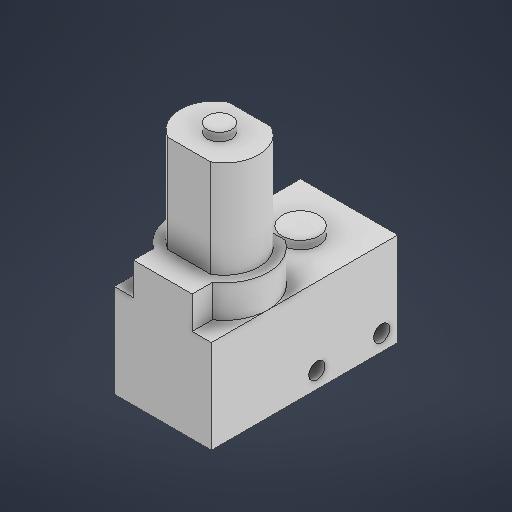
# Autodesk Inventor part: Encoder Motor
Saved by Autodesk Inventor 2026.1 (Build 301233020, 233B)
## iProperties
Created: 2025-10-23
Part Number: Encoder Motor
Material: Generic
Document SubType Name: Modeling
Designer: Asus
Density: 1 g/cm^3
Appearance: Default
Author: Asus
Autodesk Inventor part; units mm, degrees
ref_plane "YZ Plane" through (0, 0, 0) normal (1, 0, 0) x (0, 1, 0)
ref_plane "XZ Plane" through (0, 0, 0) normal (0, 1, 0) x (-1, 0, 0)
ref_plane "XY Plane" through (0, 0, 0) normal (0, 0, 1) x (1, 0, 0)
sketch "Sketch1" plane through (0, 0, 0) normal (0, 1, 0) x (-1, 0, 0)
  line L0 (0, 0) -> (-24, 0)
  line L1 (-24, 0) -> (-24, -46)
  line L2 (-24, -46) -> (0, -46)
  line L3 (0, -46) -> (0, 0)
  dimension "d0" = 24
  dimension "d1" = 46
  constraints: 8 end point, 2 parallel, 1 coincident, 1 horizontal, 1 perpendicular
  measures "d0" distance of L2.end L1.end
  measures "d1" distance of L1.end L0.end
extrude "Extrusion1" add sketch "Sketch1" along normal blind 23
sketch "Sketch2" plane through (0, 23, 0) normal (0, 1, 0) x (1, 0, 0)
  line L0 (4.75, 0) -> (19.25, 0)
  line L1 (19.25, 0) -> (19.25, 5)
  line L2 (19.25, 23) -> (4.75, 23)
  line L3 (4.75, 5) -> (4.75, 0)
  line L4 (4.75, 0) -> (19.25, 23) construction
  line L5 (19.25, 0) -> (4.75, 23) construction
  line L6 (0, 0) -> (24, 0) projected
  arc A0 (13, 23) -> (11, 23) centre (12, 23) ccw
  arc A1 (4.75, 23) -> (4.75, 5) centre (10.9013, 14) ccw
  line L7 (0, 46) -> (0, 0) projected
  arc A2 (19.25, 5) -> (19.25, 23) centre (13.0987, 14) ccw
  line L8 (24, 0) -> (24, 46) projected
  circle A3 centre (12, 34) radius 4.5
  line L9 (24, 46) -> (0, 46) projected
  point P0 (12, 11.5)
  point P1 (12, 0)
  dimension "d4" = 14.5
  dimension "d5" = 23
  dimension "d6" = 2
  dimension "d8" = 9
  dimension "d9" = 12
  constraints: 12 end point, 6 point on circle, 5 midpoint, 4 centre point, 2 parallel, 2 point on line, 2 tangent, 1 horizontal, 1 perpendicular
  measures "d4" distance of L2.end L2.start
  measures "d5" distance of L2.start L0.end
  measures "d6" diameter of A0
  measures "d8" diameter of A3
  measures "d9" distance from line of L9 A3.centre
extrude "Extrusion2" add sketch "Sketch2" along normal blind 2 contours A0 L2 | A3
extrude "Extrusion3" add sketch "Sketch2" along normal blind 8 contours L3 A1 L2 A2 L1 L0
sketch "Sketch3" plane through (0, 31, 0) normal (0, 1, 0) x (1, 0, 0)
  line L0 (17.25, 6.5) -> (6.75, 6.5)
  line L1 (6.75, 21.5) -> (17.25, 21.5)
  line L2 (17.25, 6.5) -> (6.75, 21.5) construction
  line L3 (6.75, 6.5) -> (17.25, 21.5) construction
  line L4 (19.25, 23) -> (4.75, 23) projected
  arc A0 (6.75, 21.5) -> (6.75, 6.5) centre (10.8385, 14) ccw
  arc A1 (17.25, 6.5) -> (17.25, 21.5) centre (13.1615, 14) ccw
  point P0 (0, 0)
  point P1 (12, 14)
  dimension "d17" = 8.542
  dimension "d18" = 8.542
  constraints: 8 end point, 4 point on circle, 2 centre point, 2 midpoint, 1 horizontal, 1 parallel
  measures "d17" radius of A0
  measures "d18" radius of A1
extrude "Extrusion4" add sketch "Sketch3" along normal blind 24
sketch "Sketch4" plane through (0, 55, 0) normal (0, 1, 0) x (1, 0, 0)
  circle A0 centre (12, 14) radius 3
  line L0 (17.25, 21.5) -> (6.75, 21.5) projected
  line L1 (6.75, 6.5) -> (17.25, 6.5) projected
  point P0 (0, 0)
  dimension "d21" = 6
  dimension "d22" = 7.5
  dimension "d23" = 15
  constraints: 1 centre point
  measures "d21" diameter of A0
  measures "d22" distance from line of L0 A0.centre
  measures "d23" distance between parallel lines of L0 L1
extrude "Extrusion5" add sketch "Sketch4" along normal blind 2
sketch "Sketch5" plane through (24, 0, 0) normal (1, 0, 0) x (0, 0, -1)
  circle A0 centre (42, 4) radius 2
  line L0 (46, 0) -> (46, 23) projected
  line L1 (0, 0) -> (46, 0) projected
  circle A1 centre (26, 4) radius 2
  dimension "d26" = 4
  dimension "d27" = 4
  dimension "d28" = 4
  dimension "d29" = 4
  dimension "d30" = 16
  constraints: 2 centre point
  measures "d26" diameter of A0
  measures "d27" distance from line of L0 A0.centre
  measures "d28" distance from line of L1 A0.centre
  measures "d29" diameter of A1
  measures "d30" distance of A0.centre A1.centre
extrude "Extrusion6" cut sketch "Sketch5" against normal blind 10
sketch "Sketch6" plane through (0, 0, -46) normal (-1, 0, 0) x (0, 0, 1)
  circle A0 centre (4, 4) radius 2 projected
  circle A1 centre (4, 4) radius 2
  circle A2 centre (20, 4) radius 2 projected
  circle A3 centre (20, 4) radius 2
  point P0 (46, 0)
  constraints: 2 centre point, 2 coincident
extrude "Extrusion7" cut sketch "Sketch6" against normal blind 10
sketch "Sketch7" plane through (0, 0, 0) normal (0, -1, 0) x (1, 0, 0)
  circle A0 centre (20, -10) radius 2
  line L0 (24, 0) -> (24, -46) projected
  line L1 (0, 0) -> (24, 0) projected
  circle A1 centre (4, -10) radius 2
  line L2 (0, -46) -> (0, 0) projected
  circle A2 centre (12, -34) radius 2.5
  line L3 (24, -46) -> (0, -46) projected
  point P0 (12, -46)
  dimension "d35" = 4
  dimension "d36" = 4
  dimension "d37" = 10
  dimension "d38" = 4
  dimension "d39" = 4
  dimension "d40" = 5
  dimension "d41" = 12
  constraints: 3 centre point, 1 midpoint
  measures "d35" diameter of A0
  measures "d36" distance from line of L0 A0.centre
  measures "d37" distance from line of L1 A0.centre
  measures "d38" diameter of A1
  measures "d39" distance from line of L2 A1.centre
  measures "d40" diameter of A2
  measures "d41" distance of point (12, -46) A2.centre
extrude "Extrusion8" cut sketch "Sketch7" against normal blind 10 contours A0 | A1
extrude "Extrusion9" add sketch "Sketch7" along normal blind 2 contours A2
sketch "Sketch8" plane through (12, -2, -34) normal (0, -1, 0) x (1, 0, 0)
  circle A0 centre (0, 0) radius 2.5 projected
  line L0 (1.75, -1.7854) -> (-1.75, -1.7854)
  line L1 (-1.75, -1.7854) -> (-1.75, 1.7854)
  line L2 (-1.75, 1.7854) -> (1.75, 1.7854)
  line L3 (1.75, 1.7854) -> (1.75, -1.7854)
  line L4 (1.75, -1.7854) -> (-1.75, 1.7854) construction
  line L5 (-1.75, -1.7854) -> (1.75, 1.7854) construction
  arc A1 (-1.75, -1.7854) -> (1.75, -1.7854) centre (0, 0) ccw
  arc A2 (1.75, 1.7854) -> (-1.75, 1.7854) centre (0, 0) ccw
  point P0 (-12, 34)
  point P1 (-1.75, -1.7854)
  point P2 (1.75, 1.7854)
  dimension "d46" = 3.5
  dimension "d47" = 3.5707
  constraints: 12 end point, 5 point on circle, 2 centre point, 2 concentric, 2 midpoint, 2 parallel, 1 horizontal, 1 perpendicular
  measures "d46" distance of L1.end L2.end
  measures "d47" distance between parallel lines of L2 L0
extrude "Extrusion10" add sketch "Sketch8" along normal blind 7 contours L2 A0 | L3 L0 L1 L2 | A0 L0
body "Solid1"
